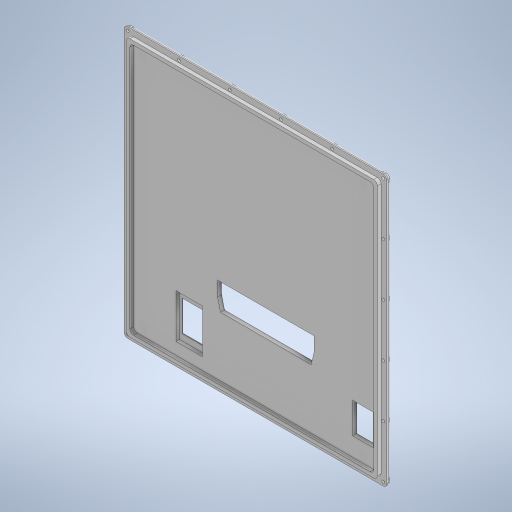
# Autodesk Inventor part: top
Saved by Autodesk Inventor 2024 (Build 280153000, 153)
## iProperties
Created: 2023-05-26
Part Number: top
Material: Generic
Document SubType Name: Modeling
Designer: elect
Density: 1 g/cm^3
Appearance: Default
Author: elect
Autodesk Inventor part; units mm, degrees
ref_plane "YZ Plane" through (0, 0, 0) normal (1, 0, 0) x (0, 1, 0)
ref_plane "XZ Plane" through (0, 0, 0) normal (0, 1, 0) x (-1, 0, 0)
ref_plane "XY Plane" through (0, 0, 0) normal (0, 0, 1) x (1, 0, 0)
sketch "Sketch1" plane through (0, 0, 0) normal (0, 0, 1) x (1, 0, 0)
  line L0 (-95.0021, 142.819) -> (127.2479, 142.819)
  line L1 (130.4229, 139.644) -> (130.4229, -88.956)
  line L2 (127.2479, -92.131) -> (-95.0021, -92.131)
  line L3 (-98.1771, -88.956) -> (-98.1771, 139.644)
  arc A0 (-95.0021, 142.819) -> (-98.1771, 139.644) centre (-95.0021, 139.644) ccw
  arc A1 (-98.1771, -88.956) -> (-95.0021, -92.131) centre (-95.0021, -88.956) ccw
  arc A2 (127.2479, -92.131) -> (130.4229, -88.956) centre (127.2479, -88.956) ccw
  arc A3 (130.4229, 139.644) -> (127.2479, 142.819) centre (127.2479, 139.644) ccw
  point P0 (0, 0)
  point P1 (130.4229, -92.131)
  point P2 (130.4229, 142.819)
  point P3 (-98.1771, -92.131)
  dimension "d0" = 228.6
  dimension "d1" = 234.95
  dimension "d2" = 3.175
  constraints: 8 end point, 8 point on circle, 8 tangent, 6 point on line, 4 centre point, 3 equal radius, 2 parallel, 1 horizontal, 1 perpendicular
  measures "d0" distance of point (130.423, -92.131) point (-98.177, -92.131)
  measures "d1" distance of point (130.423, 142.819) point (130.423, -92.131)
  measures "d2" radius of A0
extrude "Extrusion1" add sketch "Sketch1" along normal blind 4.064
sketch "Sketch3" plane through (0, 0, 4.064) normal (0, 0, 1) x (1, 0, 0)
  line L0 (-89.9221, 137.739) -> (122.1679, 137.739)
  line L1 (125.3429, 134.564) -> (125.3429, -83.876)
  line L2 (122.1679, -87.051) -> (-89.9221, -87.051)
  line L3 (-93.0971, -83.876) -> (-93.0971, 134.564)
  line L4 (127.2479, 142.819) -> (-95.0021, 142.819) projected
  line L5 (-95.0021, -92.131) -> (127.2479, -92.131) projected
  line L6 (130.4229, -88.956) -> (130.4229, 139.644) projected
  line L7 (-98.1771, 139.644) -> (-98.1771, -88.956) projected
  arc A0 (-89.9221, 137.739) -> (-93.0971, 134.564) centre (-89.9221, 134.564) ccw
  arc A1 (125.3429, 134.564) -> (122.1679, 137.739) centre (122.1679, 134.564) ccw
  arc A2 (122.1679, -87.051) -> (125.3429, -83.876) centre (122.1679, -83.876) ccw
  arc A3 (-93.0971, -83.876) -> (-89.9221, -87.051) centre (-89.9221, -83.876) ccw
  line L8 (-86.7471, 134.564) -> (118.9929, 134.564)
  line L9 (122.1679, 131.389) -> (122.1679, -80.701)
  line L10 (118.9929, -83.876) -> (-86.7471, -83.876)
  line L11 (-89.9221, -80.701) -> (-89.9221, 131.389)
  arc A4 (-86.7471, 134.564) -> (-89.9221, 131.389) centre (-86.7471, 131.389) ccw
  arc A5 (122.1679, 131.389) -> (118.9929, 134.564) centre (118.9929, 131.389) ccw
  arc A6 (118.9929, -83.876) -> (122.1679, -80.701) centre (118.9929, -80.701) ccw
  arc A7 (-89.9221, -80.701) -> (-86.7471, -83.876) centre (-86.7471, -80.701) ccw
  point P0 (0, 0)
  point P1 (-93.0971, 25.344)
  dimension "d12" = 5.08
  dimension "d13" = 5.08
  dimension "d14" = 5.08
  dimension "d15" = 5.08
  dimension "d16" = 3.175
  dimension "d17" = 3.175
  dimension "d18" = 3.175
  dimension "d19" = 3.175
  dimension "d20" = 3.175
  dimension "d21" = 3.175
  constraints: 16 end point, 16 point on circle, 16 tangent, 8 centre point, 6 equal radius, 4 parallel, 2 horizontal, 2 perpendicular, 2 point on line, 1 midpoint
  measures "d12" distance between parallel lines of L4 L0
  measures "d13" distance between parallel lines of L5 L2
  measures "d14" distance between parallel lines of L6 L1
  measures "d15" distance between parallel lines of L7 L3
  measures "d16" radius of A0
  measures "d17" distance between parallel lines of L0 L8
  measures "d18" distance between parallel lines of L1 L9
  measures "d19" distance between parallel lines of L2 L10
  measures "d20" distance from line of L11 point (-93.097, 25.344)
  measures "d21" radius of A4
extrude "Extrusion3" add sketch "Sketch3" along normal blind 3.175
sketch "Sketch11" plane through (0, 0, 0) normal (0, 0, -1) x (-1, 0, 0)
  arc A0 (-127.2479, 142.819) -> (-130.4229, 139.644) centre (-127.2479, 139.644) ccw projected
  line L0 (89.9221, 137.739) -> (-122.1679, 137.739) projected
  line L1 (-125.3429, 134.564) -> (-125.3429, -83.876) projected
  point P0 (0, 0)
  point P1 (-82.7979, 139.644)
  point P2 (-38.3479, 139.644)
  point P3 (6.1021, 139.644)
  point P4 (50.5521, 139.644)
  point P5 (95.0021, 139.644)
  point P6 (-127.2479, 93.924)
  point P7 (-127.2479, 48.204)
  point P8 (-127.2479, 2.484)
  point P9 (-127.2479, -43.236)
  point P10 (-127.2479, -88.956)
  point P11 (-82.7979, -88.956)
  point P12 (-38.3479, -88.956)
  point P13 (6.1021, -88.956)
  point P14 (50.5521, -88.956)
  point P15 (95.0021, -88.956)
  point P16 (95.0021, -43.236)
  point P17 (95.0021, 2.484)
  point P18 (95.0021, 48.204)
  point P19 (95.0021, 93.924)
  dimension "d124" = 44.45
  dimension "d131" = 45.72
  dimension "d138" = 44.45
  dimension "d145" = 45.72
  constraints: 2 horizontal, 2 vertical, 1 coincident, 19 other
  measures "d124" distance of point (-127.248, 139.644) point (-82.798, 139.644)
  measures "d131" distance of point (-127.248, 139.644) point (-127.248, 93.924)
  measures "d138" distance of point (-127.248, -88.956) point (-82.798, -88.956)
  measures "d145" distance of point (95.002, -88.956) point (95.002, -43.236)
hole "Hole4" at (127.2479, 139.644, 0) at (82.7979, 139.644, 0) at (38.3479, 139.644, 0) at (-6.1021, 139.644, 0) at (-50.5521, 139.644, 0) at (-95.0021, 139.644, 0) at (127.2479, 93.924, 0) at (127.2479, 48.204, 0) at (127.2479, 2.484, 0) at (127.2479, -43.236, 0) at (127.2479, -88.956, 0) at (82.7979, -88.956, 0) at (38.3479, -88.956, 0) at (-6.1021, -88.956, 0) at (-50.5521, -88.956, 0) at (-95.0021, -88.956, 0) at (-95.0021, -43.236, 0) at (-95.0021, 2.484, 0) at (-95.0021, 48.204, 0) at (-95.0021, 93.924, 0) direction (0, 0, 1) diameter 2.54 end through all counterbore diameter 5.08 counterbore depth 2.54
fillet "Fillet3" radius 3.048 8 edges at (-97.2471, 141.8891, 0) (-98.1771, 25.344, 0) (-97.2471, -91.201, 0) (16.1229, -92.131, 0) (129.493, -91.201, 0) (130.4229, 25.344, 0) (129.493, 141.8891, 0) (16.1229, 142.819, 0)
sketch "Sketch12" plane through (0, 0, 0) normal (0, 0, -1) x (-1, 0, 0)
  line L0 (-67.0499, -9.073) -> (16.7701, -9.073)
  line L1 (16.7701, -9.073) -> (16.7701, -31.933)
  line L2 (16.7701, -31.933) -> (-67.0499, -31.933)
  line L3 (-67.0499, -31.933) -> (-67.0499, -9.073)
  line L4 (-127.3749, -40.6992) -> (-127.3749, -0.0528) projected
  line L5 (-40.8847, -89.083) -> (-80.2611, -89.083) projected
  line L6 (-67.0499, -21.773) -> (-64.5099, -31.933)
  line L7 (16.7701, -21.773) -> (14.2301, -31.933)
  point P0 (0, 0)
  dimension "d158" = 60.325
  dimension "d159" = 83.82
  dimension "d160" = 22.86
  dimension "d161" = 57.15
  dimension "d174" = 10.16
  dimension "d175" = 2.54
  dimension "d176" = 10.16
  dimension "d177" = 2.54
  constraints: 12 end point, 4 point on line, 2 parallel, 1 horizontal, 1 perpendicular
  measures "d158" distance between parallel lines of L4 L3
  measures "d159" distance of L0.start L0.end
  measures "d160" distance of L2.end L0.start
  measures "d161" distance between parallel lines of L5 L2
  measures "d174" distance of L1.end L7.start
  measures "d175" distance of L1.end L7.end
  measures "d176" distance of L2.end L6.start
  measures "d177" distance of L2.end L6.end
extrude "Extrusion7" cut sketch "Sketch12" against normal up to surface (4.064 mm away) contours L0 L1 L7 L2 L6 L3
sketch "Sketch13" plane through (0, 0, 0) normal (0, 0, -1) x (-1, 0, 0)
  line L0 (-118.4849, -40.823) -> (-100.7049, -40.823)
  line L1 (-100.7049, -40.823) -> (-100.7049, -67.493)
  line L2 (-100.7049, -67.493) -> (-118.4849, -67.493)
  line L3 (-118.4849, -67.493) -> (-118.4849, -40.823)
  line L4 (32.6451, -40.823) -> (50.4251, -40.823)
  line L5 (50.4251, -40.823) -> (50.4251, -67.493)
  line L6 (50.4251, -67.493) -> (32.6451, -67.493)
  line L7 (32.6451, -67.493) -> (32.6451, -40.823)
  line L8 (-85.3347, -89.083) -> (-124.7111, -89.083) projected
  line L9 (-127.3749, -86.4192) -> (-127.3749, -45.7728) projected
  line L10 (48.0153, -89.083) -> (8.6389, -89.083) projected
  point P0 (0, 0)
  point P1 (-127.3749, -66.096)
  dimension "d164" = 17.78
  dimension "d165" = 26.67
  dimension "d166" = 17.78
  dimension "d167" = 26.67
  dimension "d168" = 21.59
  dimension "d169" = 8.89
  dimension "d170" = 133.35
  dimension "d171" = 21.59
  constraints: 16 end point, 4 parallel, 2 horizontal, 2 perpendicular, 1 midpoint, 1 point on line
  measures "d164" distance of L0.start L0.end
  measures "d165" distance of L0.end L1.end
  measures "d166" distance of L4.start L4.end
  measures "d167" distance of L6.end L4.start
  measures "d168" distance between parallel lines of L8 L2
  measures "d169" distance from line of point (-127.375, -66.096) L3
  measures "d170" distance between parallel lines of L7 L1
  measures "d171" distance between parallel lines of L10 L6
extrude "Extrusion8" cut sketch "Sketch13" against normal up to surface (4.064 mm away)
sketch "Sketch15" plane through (0, 0, 4.064) normal (0, 0, 1) x (1, 0, 0)
  line L0 (-52.9651, -35.108) -> (-30.1051, -35.108)
  line L1 (-30.1051, -35.108) -> (-30.1051, -73.208)
  line L2 (-30.1051, -73.208) -> (-52.9651, -73.208)
  line L3 (-52.9651, -73.208) -> (-52.9651, -35.108)
  line L4 (-50.4251, -40.823) -> (-32.6451, -40.823) projected
  line L5 (-32.6451, -67.493) -> (-50.4251, -67.493) projected
  line L6 (-32.6451, -40.823) -> (-32.6451, -67.493) projected
  line L7 (-50.4251, -67.493) -> (-50.4251, -40.823) projected
  point P0 (0, 0)
  dimension "d186" = 5.715
  dimension "d187" = 5.715
  dimension "d188" = 2.54
  dimension "d189" = 2.54
  dimension "d190" = 22.86
  dimension "d191" = 38.1
  constraints: 8 end point, 2 parallel, 1 horizontal, 1 perpendicular
  measures "d186" distance between parallel lines of L4 L0
  measures "d187" distance between parallel lines of L2 L5
  measures "d188" distance between parallel lines of L1 L6
  measures "d189" distance between parallel lines of L3 L7
  measures "d190" distance of L0.start L0.end
  measures "d191" distance of L2.end L0.start
extrude "Extrusion10" cut sketch "Sketch15" against normal blind 2.794
fillet "Fillet4" radius 0.7937 14 edges at (25.1399, -9.073, 0) (67.0499, -15.423, 0) (65.7799, -26.853, 0) (25.1399, -31.933, 0) (-15.5001, -26.853, 0) (-16.7701, -15.423, 0) (-32.6451, -54.158, 0) (-41.5351, -40.823, 0) (-50.4251, -54.158, 0) (-41.5351, -67.493, 0) (100.7049, -54.158, 0) (109.5949, -40.823, 0) (118.4849, -54.158, 0) (109.5949, -67.493, 0)
body "Solid1"
